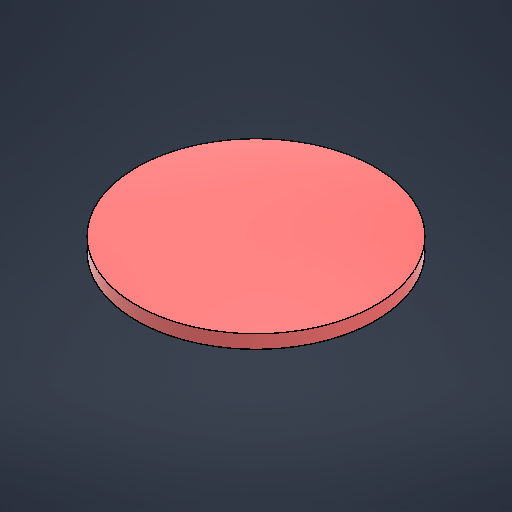
# Autodesk Inventor part: E-Stop Button
Saved by Autodesk Inventor 2026 (Build 300175050, 175E)
## iProperties
Created: 2025-06-28
Part Number: E-Stop Button
Material: ABS Plastic
Document SubType Name: Modeling
Designer: Joshua Eah
Density: 1.06 g/cm^3
Appearance: Smooth - Red
Author: Joshua Eah
Autodesk Inventor part; units mm, degrees
ref_plane "YZ Plane" through (0, 0, 0) normal (1, 0, 0) x (0, 1, 0)
ref_plane "XZ Plane" through (0, 0, 0) normal (0, 1, 0) x (-1, 0, 0)
ref_plane "XY Plane" through (0, 0, 0) normal (0, 0, 1) x (1, 0, 0)
sketch "Sketch1" plane through (0, 0, 0) normal (0, 1, 0) x (-1, 0, 0)
  circle A0 centre (0, 0) radius 11.375
  circle A1 centre (0, 0) radius 20
  circle A2 centre (0, 0) radius 18.25
  dimension "d0" = 22.75
  dimension "d1" = 40
  dimension "d2" = 36.5
  constraints: 3 centre point, 3 coincident
  measures "d0" diameter of A0
  measures "d1" diameter of A1
  measures "d2" diameter of A2
extrude "Extrusion1" add sketch "Sketch1" along normal blind 12.25 contours A0 | A1 | A2
extrude "Extrusion2" cut sketch "Sketch1" along normal blind 6 contours A1 | A2
sketch "Sketch2" plane through (0, 0, 0) normal (1, 0, 0) x (0, 1, 0)
  line L0 (6, -20) -> (6, 20) projected
  line L1 (12.25, -20) -> (12.25, 20) projected
  line L2 (6, 20) -> (12.25, 20) projected
  line L3 (12.25, -20) -> (8.25, -20)
  line L4 (8.25, -20) -> (8.25, 20)
  line L5 (8.25, 20) -> (12.25, 20)
  line L6 (12.25, 20) -> (12.25, -20)
  arc A0 (8.25, -20) -> (8.25, 20) centre (-69.846, 0) ccw
  line L7 (-50.15, 0) -> (22.65, 0) projected
  line L8 (6, -20) -> (6, 20) projected
  line L9 (6, 11.375) -> (6, -11.375) projected
  line L10 (0, 11.375) -> (0, -11.375) projected
  line L11 (6, 11.375) -> (12.25, 11.375)
  line L12 (12.25, 11.375) -> (12.25, -11.375)
  line L13 (12.25, -11.375) -> (6, -11.375)
  line L14 (6, -11.375) -> (6, 11.375)
  line L15 (0, 11.375) -> (12.25, 11.375)
  line L16 (12.25, 11.375) -> (12.25, -11.375)
  line L17 (12.25, -11.375) -> (0, -11.375)
  line L18 (0, -11.375) -> (0, 11.375)
  line L19 (8.25, 18.5) -> (6, 18.5)
  line L20 (6, 18.5) -> (6, -18.5)
  line L21 (6, -18.5) -> (8.25, -18.5)
  line L22 (8.25, -18.5) -> (8.25, 18.5)
  arc A1 (7.9022, -19.9109) -> (8.25, 18.5) centre (-69.846, 0) ccw
  point P0 (12.25, 0)
  point P1 (6, 0)
  point P2 (8.25, 0)
  point P3 (10.7703, 0)
  point P4 (12.25, 0)
  point P5 (9.6011, 11.375)
  dimension "d8" = 4
  constraints: 32 end point, 8 parallel, 4 horizontal, 4 perpendicular, 4 point on circle, 4 point on line, 2 centre point
  measures "d8" distance of L4.end L5.end
revolve "Revolution1" cut sketch "Sketch2" angle 360 about axis through (0, -10, 0) along (0, 1, 0) contours L0 L19 L4 L11 | L4 A1 L11 | A0 L11 L1 L7 | A0 L2 L1 L11
sketch "Sketch3" plane through (0, 0, 0) normal (0, -1, 0) x (1, 0, 0)
  circle A0 centre (0, 0) radius 11.375 projected
hole "Hole1" at (0, 0, 0) direction (0, 1, 0) diameter 17.1881 depth 5 thread size "M18x0.75" class "6H" standard "ANSI Metric M Profile"
body "Solid1"
